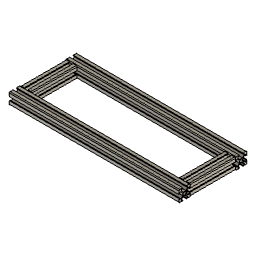
Aluminum Frame v1 (Autodesk Fusion 360 design; units mm, degrees)
Autodesk Fusion 360 part; units mm, degrees
sketch "Sketch1" plane through (0, 0, 0) normal (0, 0, 1) x (1, 0, 0)
  line L0 (-150, 50) -> (150, 50)
  line L1 (150, 50) -> (150, -50) construction
  line L2 (150, -50) -> (-150, -50)
  line L3 (-150, -50) -> (-150, 50) construction
  line L4 (-150, 50) -> (150, -50) construction
  line L5 (150, 50) -> (-150, -50) construction
  line L6 (-140, 40) -> (-140, -40)
  dimension "d1" = 300
  dimension "d2" = 100
  dimension "d3" = 10
  dimension "d4" = 10
  dimension "d5" = 80
  constraint horizontal L0
  constraint perpendicular L0 L1
  constraint parallel L0 L2
  constraint parallel L1 L3
  constraint coincident L4 origin
  constraint coincident L5 origin
  constraint vertical L6
  measures "d1" distance of L1.end L2.end
  measures "d2" distance of L0.end L1.end
  measures "d3" vertical distance of L2.end L6.end
  measures "d4" distance of L3 L6
  measures "d5" distance of L6.start L6.end
ref_plane "WorkPlane1" through (0, -50, 0) normal (-1, 0, 0) x (0, -1, 0)
sketch "Sketch2" plane through (0, -50, 0) normal (-1, 0, 0) x (0, -1, 0)
  line L0 (0, 3.1) -> (2.25, 3.1)
  line L1 (2.25, 3.1) -> (5.5, 6.35)
  line L2 (5.5, 6.35) -> (5.5, 8.5)
  line L3 (5.5, 8.5) -> (3.1, 8.5)
  line L4 (3.1, 8.5) -> (3.1, 10)
  line L5 (3.1, 10) -> (8.5, 10)
  arc A0 (10, 8.5) -> (8.5, 10) centre (8.5, 8.5) ccw
  line L6 (3.1, 0) -> (3.1, 2.25)
  line L7 (3.1, 2.25) -> (6.35, 5.5)
  line L8 (6.35, 5.5) -> (8.5, 5.5)
  line L9 (8.5, 5.5) -> (8.5, 3.1)
  line L10 (8.5, 3.1) -> (10, 3.1)
  line L11 (10, 3.1) -> (10, 8.5)
  line L12 (0, 3.1) -> (-2.25, 3.1)
  line L13 (-2.25, 3.1) -> (-5.5, 6.35)
  line L14 (-5.5, 6.35) -> (-5.5, 8.5)
  line L15 (-5.5, 8.5) -> (-3.1, 8.5)
  line L16 (-3.1, 8.5) -> (-3.1, 10)
  line L17 (-3.1, 10) -> (-8.5, 10)
  arc A1 (-8.5, 10) -> (-10, 8.5) centre (-8.5, 8.5) ccw
  line L18 (-3.1, 0) -> (-3.1, 2.25)
  line L19 (-3.1, 2.25) -> (-6.35, 5.5)
  line L20 (-6.35, 5.5) -> (-8.5, 5.5)
  line L21 (-8.5, 5.5) -> (-8.5, 3.1)
  line L22 (-8.5, 3.1) -> (-10, 3.1)
  line L23 (-10, 3.1) -> (-10, 8.5)
  line L24 (0, -3.1) -> (-2.25, -3.1)
  line L25 (-2.25, -3.1) -> (-5.5, -6.35)
  line L26 (-5.5, -6.35) -> (-5.5, -8.5)
  line L27 (-5.5, -8.5) -> (-3.1, -8.5)
  line L28 (-3.1, -8.5) -> (-3.1, -10)
  line L29 (-3.1, -10) -> (-8.5, -10)
  arc A2 (-10, -8.5) -> (-8.5, -10) centre (-8.5, -8.5) ccw
  line L30 (-3.1, 0) -> (-3.1, -2.25)
  line L31 (-3.1, -2.25) -> (-6.35, -5.5)
  line L32 (-6.35, -5.5) -> (-8.5, -5.5)
  line L33 (-8.5, -5.5) -> (-8.5, -3.1)
  line L34 (-8.5, -3.1) -> (-10, -3.1)
  line L35 (-10, -3.1) -> (-10, -8.5)
  line L36 (0, -3.1) -> (2.25, -3.1)
  line L37 (2.25, -3.1) -> (5.5, -6.35)
  line L38 (5.5, -6.35) -> (5.5, -8.5)
  line L39 (5.5, -8.5) -> (3.1, -8.5)
  line L40 (3.1, -8.5) -> (3.1, -10)
  line L41 (3.1, -10) -> (8.5, -10)
  arc A3 (8.5, -10) -> (10, -8.5) centre (8.5, -8.5) ccw
  line L42 (3.1, 0) -> (3.1, -2.25)
  line L43 (3.1, -2.25) -> (6.35, -5.5)
  line L44 (6.35, -5.5) -> (8.5, -5.5)
  line L45 (8.5, -5.5) -> (8.5, -3.1)
  line L46 (8.5, -3.1) -> (10, -3.1)
  line L47 (10, -3.1) -> (10, -8.5)
  circle A4 centre (0, 0) radius 2.5
ref_plane "WorkPlane2" through (-140, 0, 0) normal (0, -1, 0) x (1, 0, 0)
sketch "Sketch3" plane through (-140, 0, 0) normal (0, -1, 0) x (1, 0, 0)
  line L0 (0, 3.1) -> (2.25, 3.1)
  line L1 (2.25, 3.1) -> (5.5, 6.35)
  line L2 (5.5, 6.35) -> (5.5, 8.5)
  line L3 (5.5, 8.5) -> (3.1, 8.5)
  line L4 (3.1, 8.5) -> (3.1, 10)
  line L5 (3.1, 10) -> (8.5, 10)
  arc A0 (10, 8.5) -> (8.5, 10) centre (8.5, 8.5) ccw
  line L6 (3.1, 0) -> (3.1, 2.25)
  line L7 (3.1, 2.25) -> (6.35, 5.5)
  line L8 (6.35, 5.5) -> (8.5, 5.5)
  line L9 (8.5, 5.5) -> (8.5, 3.1)
  line L10 (8.5, 3.1) -> (10, 3.1)
  line L11 (10, 3.1) -> (10, 8.5)
  line L12 (0, 3.1) -> (-2.25, 3.1)
  line L13 (-2.25, 3.1) -> (-5.5, 6.35)
  line L14 (-5.5, 6.35) -> (-5.5, 8.5)
  line L15 (-5.5, 8.5) -> (-3.1, 8.5)
  line L16 (-3.1, 8.5) -> (-3.1, 10)
  line L17 (-3.1, 10) -> (-8.5, 10)
  arc A1 (-8.5, 10) -> (-10, 8.5) centre (-8.5, 8.5) ccw
  line L18 (-3.1, 0) -> (-3.1, 2.25)
  line L19 (-3.1, 2.25) -> (-6.35, 5.5)
  line L20 (-6.35, 5.5) -> (-8.5, 5.5)
  line L21 (-8.5, 5.5) -> (-8.5, 3.1)
  line L22 (-8.5, 3.1) -> (-10, 3.1)
  line L23 (-10, 3.1) -> (-10, 8.5)
  line L24 (0, -3.1) -> (-2.25, -3.1)
  line L25 (-2.25, -3.1) -> (-5.5, -6.35)
  line L26 (-5.5, -6.35) -> (-5.5, -8.5)
  line L27 (-5.5, -8.5) -> (-3.1, -8.5)
  line L28 (-3.1, -8.5) -> (-3.1, -10)
  line L29 (-3.1, -10) -> (-8.5, -10)
  arc A2 (-10, -8.5) -> (-8.5, -10) centre (-8.5, -8.5) ccw
  line L30 (-3.1, 0) -> (-3.1, -2.25)
  line L31 (-3.1, -2.25) -> (-6.35, -5.5)
  line L32 (-6.35, -5.5) -> (-8.5, -5.5)
  line L33 (-8.5, -5.5) -> (-8.5, -3.1)
  line L34 (-8.5, -3.1) -> (-10, -3.1)
  line L35 (-10, -3.1) -> (-10, -8.5)
  line L36 (0, -3.1) -> (2.25, -3.1)
  line L37 (2.25, -3.1) -> (5.5, -6.35)
  line L38 (5.5, -6.35) -> (5.5, -8.5)
  line L39 (5.5, -8.5) -> (3.1, -8.5)
  line L40 (3.1, -8.5) -> (3.1, -10)
  line L41 (3.1, -10) -> (8.5, -10)
  arc A3 (8.5, -10) -> (10, -8.5) centre (8.5, -8.5) ccw
  line L42 (3.1, 0) -> (3.1, -2.25)
  line L43 (3.1, -2.25) -> (6.35, -5.5)
  line L44 (6.35, -5.5) -> (8.5, -5.5)
  line L45 (8.5, -5.5) -> (8.5, -3.1)
  line L46 (8.5, -3.1) -> (10, -3.1)
  line L47 (10, -3.1) -> (10, -8.5)
  circle A4 centre (0, 0) radius 2.5
sweep "Sweep1" add profiles "Sketch3" path "Sketch1" along L6 section 1 makes body 1
sweep "Sweep2" add profiles "Sketch2" path "Sketch1" along L2 section 1 separate body makes body 2
mirror "Mirror1" about plane through (0, 0, 0) normal (1, 0, 0) of bodies 1 makes body 3
mirror "Mirror2" about plane through (0, 0, 0) normal (0, 1, 0) of bodies 2 makes body 4
